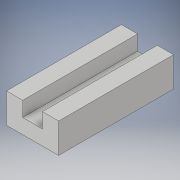
# Autodesk Inventor part: Rail Slider
Saved by Autodesk Inventor 2017 (Build 210142000, 142)
## iProperties
Created: 2017-05-04
Part Number: Rail Slider
Material: Generic
Document SubType Name: Modeling
Designer: Jon
Density: 1 g/cm^3
Appearance: Default
Author: Jon
Autodesk Inventor part; units mm, degrees
ref_plane "YZ Plane" through (0, 0, 0) normal (1, 0, 0) x (0, 1, 0)
ref_plane "XZ Plane" through (0, 0, 0) normal (0, 1, 0) x (-1, 0, 0)
ref_plane "XY Plane" through (0, 0, 0) normal (0, 0, 1) x (1, 0, 0)
sketch "Sketch1" plane through (0, 0, 0) normal (0, 0, 1) x (1, 0, 0)
  line L0 (7.6927, 4.9102) -> (7.6927, -20.4898)
  line L1 (7.6927, -20.4898) -> (-36.7573, -20.4898)
  line L2 (-36.7573, -20.4898) -> (-36.7573, 4.9102)
  line L3 (-6.1503, 2.7687) -> (-6.1503, -7.7898)
  line L4 (-6.1503, -7.7898) -> (-22.9143, -7.7898)
  line L5 (-22.9143, -7.7898) -> (-22.9143, 2.7687)
  line L6 (-22.9143, 2.7687) -> (-22.9143, 4.9102)
  line L7 (-6.1503, 2.7687) -> (-6.1503, 4.9102)
  line L8 (-36.7573, 4.9102) -> (-22.9143, 4.9102)
  line L9 (-6.1503, 4.9102) -> (7.6927, 4.9102)
  point P0 (0, 0)
  dimension "d0" = 44.45
  dimension "d1" = 25.4
  dimension "d2" = 16.764
  dimension "d4" = 13.843
  dimension "d5" = 13.843
  dimension "d6" = 12.7
  constraints: 20 end point, 6 perpendicular, 4 parallel, 2 horizontal
  measures "d0" distance of L2.end L0.start
  measures "d1" distance of L0.start L0.end
  measures "d2" distance of L3.end L4.end
  measures "d4" distance between parallel lines of L2 L5
  measures "d5" distance between parallel lines of L0 L3
  measures "d6" distance between parallel lines of L1 L4
extrude "Extrusion1" add sketch "Sketch1" along normal blind 97.917
sketch "Sketch2" plane through (-36.7573, -20.4898, 0) normal (0, -1, 0) x (1, 0, 0)
  line L0 (44.45, 0) -> (44.45, 97.917) projected
  line L1 (0, 0) -> (0, 97.917) projected
  line L2 (0, 0) -> (44.45, 0) projected
  line L3 (0, 97.917) -> (44.45, 97.917) projected
  point P0 (36.7573, 0)
  point P1 (38.6715, 22.225)
  point P2 (5.7785, 22.225)
  point P3 (5.7785, 75.692)
  point P4 (38.6715, 75.692)
  dimension "d9" = 5.7785
  dimension "d10" = 5.7785
  dimension "d11" = 22.225
  dimension "d12" = 22.225
  dimension "d13" = 5.7785
  dimension "d14" = 5.7785
  dimension "d15" = 22.225
  dimension "d16" = 22.225
  dimension "d17" = 53.467
  dimension "d18" = 53.467
  measures "d9" distance from line of L0 point (38.671, 22.225)
  measures "d10" distance from line of L1 point (5.778, 22.225)
  measures "d11" distance from line of L2 point (38.671, 22.225)
  measures "d12" distance from line of L2 point (5.778, 22.225)
  measures "d13" distance from line of L1 point (5.778, 75.692)
  measures "d14" distance from line of L0 point (38.671, 75.692)
  measures "d15" distance from line of L3 point (5.778, 75.692)
  measures "d16" distance from line of L3 point (38.671, 75.692)
  measures "d17" distance of point (5.778, 22.225) point (5.778, 75.692)
  measures "d18" distance of point (38.671, 22.225) point (38.671, 75.692)
hole "Hole1" at (1.9142, -20.4898, 22.225) at (-30.9788, -20.4898, 22.225) at (-30.9788, -20.4898, 75.692) at (1.9142, -20.4898, 75.692) direction (0, 1, 0) diameter 3.81 depth 7.62
equation "\"d10\" = d9"
equation "\"d12\" = d11"
equation "\"d13\" = d9"
equation "\"d14\" = d9"
equation "\"d15\" = d11"
equation "\"d16\" = d11"
body "Solid1"
